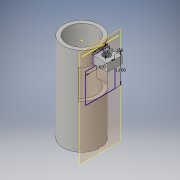
# Autodesk Inventor part: MainBody
Saved by Autodesk Inventor 2016 (Build 200138000, 138)
## iProperties
Created: 2016-03-07
Part Number: MainBody
Material: Generic
Document SubType Name: Modeling
Designer: yash
Density: 1 g/cm^3
Appearance: Default
Author: yash
Autodesk Inventor part; units mm, degrees
note: some values were not read from the file. Chosen so that the rebuilt part matches the saved one: direction of "Hole1".
ref_plane "XZ Plane" through (0, 0, 0) normal (0, 1, 0) x (-1, 0, 0)
ref_plane "XY Plane" through (0, 0, 0) normal (0, 0, 1) x (1, 0, 0)
sketch "Sketch1" plane through (0, 0, 0) normal (0, 1, 0) x (-1, 0, 0)
  circle A0 centre (0, 0) radius 12.7
  circle A1 centre (0, 0) radius 15.875
  dimension "d0" = 25.4
  dimension "d1" = 3.175
  constraints: 2 centre point, 2 coincident
  measures "d0" diameter of A0
  measures "d1" radial gap between concentric circles of A1 A0
extrude "Extrusion1" add sketch "Sketch1" along normal blind 76.2
ref_plane "Work Plane1" through (15.875, 0, 0) normal (1, 0, 0) x (0, 1, 0)
sketch "Sketch2" plane through (15.875, 0, 0) normal (1, 0, 0) x (0, 1, 0)
  line L0 (63.5, 12.7) -> (38.1, 12.7)
  line L1 (38.1, 12.7) -> (38.1, -12.7)
  line L2 (38.1, -12.7) -> (63.5, -12.7)
  line L3 (63.5, -12.7) -> (63.5, 12.7)
  line L4 (76.2, -15.875) -> (76.2, 15.875) projected
  line L5 (72.39, 6.35) -> (66.04, 6.35)
  line L6 (66.04, 6.35) -> (66.04, -6.35)
  line L7 (66.04, -6.35) -> (72.39, -6.35)
  line L8 (72.39, -6.35) -> (72.39, 6.35)
  point P0 (0, 0)
  point P1 (63.5, 0)
  point P2 (66.04, 0)
  dimension "d4" = 25.4
  dimension "d5" = 25.4
  dimension "d6" = 12.7
  dimension "d7" = 2.54
  dimension "d8" = 6.35
  dimension "d13" = 12.7
  constraints: 16 end point, 4 parallel, 2 horizontal, 2 horizontal alignment, 2 midpoint, 2 perpendicular
  measures "d4" distance of L2.end L0.start
  measures "d5" distance of L1.end L2.end
  measures "d6" distance between parallel lines of L3 L4
  measures "d7" distance between parallel lines of L3 L6
  measures "d8" distance of L6.end L7.end
  measures "d13" distance of L7.end L5.start
extrude "Extrusion2" cut sketch "Sketch2" against normal up to next contours L3 L2 L1 L0
extrude "Extrusion3" add sketch "Sketch2" along normal blind 12.7 contours L8 L7 L6 L5
sketch "Sketch3" plane through (15.875, 72.39, 0) normal (0, 1, 0) x (1, 0, 0)
  point P0 (-15.875, 0)
extrude "Extrusion4" add sketch "Sketch2" against normal up to next contours L8 L7 L6 L5
sketch "Sketch4" plane through (14.5497, 72.39, 6.35) normal (0, 1, 0) x (1, 0, 0)
  line L0 (0, 12.7) -> (14.0253, 12.7) projected
  line L1 (14.0253, 12.7) -> (14.0253, 0) projected
  point P0 (-14.5497, 6.35)
  point P1 (7.0127, 6.35)
  point P2 (7.0127, 12.7)
  point P3 (14.0253, 6.35)
  constraints: 2 midpoint, 1 horizontal alignment, 1 vertical alignment
hole "Hole1" at (21.5623, 72.39, 0) direction (0, -1, 0) diameter 6.35 end up to surface
body "Solid1"
